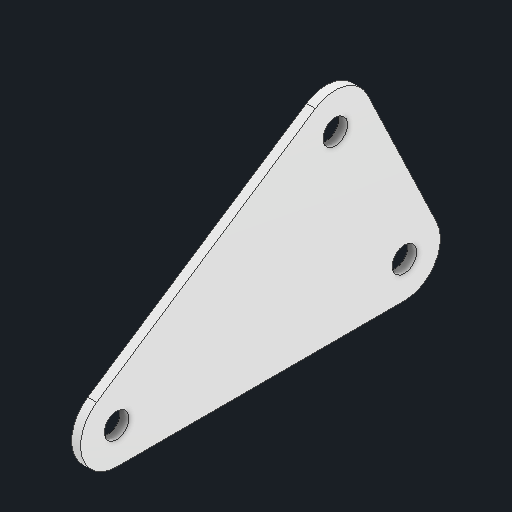
# Autodesk Inventor part: Conveyer Gusset
Saved by Autodesk Inventor 2025 (Build 290162000, 162)
## iProperties
Created: 2024-12-31
Part Number: Conveyer Gusset
Material: Acetal Resin, White
Document SubType Name: Modeling
Designer: Averey Ku
Density: 1.425 g/cm^3
Appearance: Smooth - White
Author: Averey Ku
Autodesk Inventor part; units mm, degrees
ref_plane "YZ Plane" through (0, 0, 0) normal (1, 0, 0) x (0, 1, 0)
ref_plane "XZ Plane" through (0, 0, 0) normal (0, 1, 0) x (-1, 0, 0)
ref_plane "XY Plane" through (0, 0, 0) normal (0, 0, 1) x (1, 0, 0)
sketch "Sketch1" plane through (0, 0, 0) normal (1, 0, 0) x (0, 1, 0)
  circle A0 centre (-11.1881, 27.3725) radius 2.1844
  circle A1 centre (-11.1881, -23.4275) radius 2.1844
  circle A2 centre (14.4132, -11.2197) radius 2.1844
  arc A3 (17.1463, -16.9515) -> (19.7048, -7.7094) centre (14.4132, -11.2197) ccw
  arc A4 (-17.5381, -23.4275) -> (-8.455, -29.1592) centre (-11.1881, -23.4275) ccw
  arc A5 (-5.8966, 30.8828) -> (-17.5381, 27.3725) centre (-11.1881, 27.3725) ccw
  line L0 (-5.8966, 30.8828) -> (19.7048, -7.7094)
  line L1 (17.1463, -16.9515) -> (-8.455, -29.1592)
  line L2 (-17.5381, -23.4275) -> (-17.5381, 27.3725)
  point P0 (0, 0)
  dimension "d0" = 12.7
  dimension "d1" = 12.7
  dimension "d2" = 12.7
  constraints: 6 centre point, 6 end point, 6 point on circle, 6 tangent, 3 coincident, 7 other
  measures "d0" diameter of A3
  measures "d1" diameter of A4
  measures "d2" diameter of A5
extrude "Extrusion1" add sketch "Sketch1" along normal blind 1.5875
body "Solid1"
